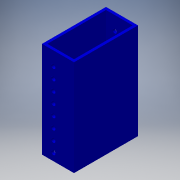
# Autodesk Inventor part: 2018 Scissor Standoff Iner
Saved by Autodesk Inventor 2018 (Build 220112000, 112)
## iProperties
Created: 2018-01-26
Part Number: 2018 Scissor Standoff Iner
Material: Generic
Document SubType Name: Modeling
Designer: Apple
Density: 1 g/cm^3
Appearance: Default
Author: Apple
Autodesk Inventor part; units mm, degrees
ref_plane "YZ Plane" through (0, 0, 0) normal (1, 0, 0) x (0, 1, 0)
ref_plane "XZ Plane" through (0, 0, 0) normal (0, 1, 0) x (-1, 0, 0)
ref_plane "XY Plane" through (0, 0, 0) normal (0, 0, 1) x (1, 0, 0)
sketch "Sketch1" plane through (0, 0, 0) normal (0, 1, 0) x (-1, 0, 0)
  line L0 (-158.7435, 10.9468) -> (-196.8435, 10.9468)
  line L1 (-196.8435, 10.9468) -> (-196.8435, 87.1468)
  line L2 (-196.8435, 87.1468) -> (-158.7435, 87.1468)
  line L3 (-158.7435, 87.1468) -> (-158.7435, 10.9468)
  line L4 (-161.9185, 83.9718) -> (-193.6685, 83.9718)
  line L5 (-193.6685, 83.9718) -> (-193.6685, 14.1218)
  line L6 (-193.6685, 14.1218) -> (-161.9185, 14.1218)
  line L7 (-161.9185, 14.1218) -> (-161.9185, 83.9718)
  point P0 (0, 0)
  dimension "d0" = 76.2
  dimension "d1" = 38.1
  dimension "d2" = 3.175
  constraints: 16 end point, 4 parallel, 2 perpendicular, 1 horizontal, 3 other
  measures "d0" distance of L0.end L1.end
  measures "d1" distance of L1.end L2.end
  measures "d2" distance between parallel lines of L2 L4
extrude "Extrusion1" add sketch "Sketch1" along normal blind 114.3
sketch "Sketch2" plane through (158.7435, 0, 87.1468) normal (0, 0, 1) x (1, 0, 0)
  line L0 (0, 0) -> (0, 114.3) projected
  line L1 (38.1, 0) -> (0, 0) projected
  point P0 (-158.7435, 0)
  point P1 (13.46, 8.89)
  point P2 (13.46, 21.59)
  point P3 (13.46, 34.29)
  point P4 (13.46, 46.99)
  point P5 (13.46, 59.69)
  point P6 (13.46, 72.39)
  point P7 (13.46, 85.09)
  point P8 (13.46, 97.79)
  dimension "d5" = 13.46
  dimension "d6" = 8.89
  dimension "d9" = 12.7
  constraints: 1 vertical, 7 other
  measures "d5" distance from line of point (13.46, 8.89) L0
  measures "d6" distance from line of L1 point (13.46, 8.89)
  measures "d9" distance of point (13.46, 8.89) point (13.46, 21.59)
hole "Hole1" at (172.2035, 8.89, 87.1468) at (172.2035, 21.59, 87.1468) at (172.2035, 34.29, 87.1468) at (172.2035, 46.99, 87.1468) at (172.2035, 59.69, 87.1468) at (172.2035, 72.39, 87.1468) at (172.2035, 85.09, 87.1468) at (172.2035, 97.79, 87.1468) direction (0, 0, -1) diameter 5.08 end through all
body "Solid1"
